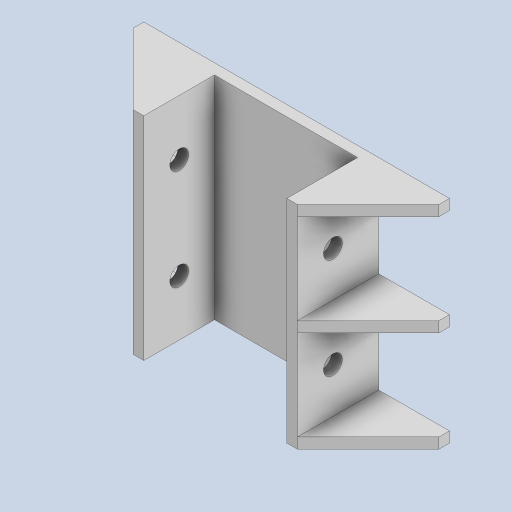
# Autodesk Inventor part: 2040 psu adapter
Saved by Autodesk Inventor 2024 (Build 280153000, 153)
## iProperties
Created: 2025-04-07
Part Number: 2040 psu adapter
Material: Generic
Document SubType Name: Modeling
Designer: jp.reyesf
Density: 1 g/cm^3
Appearance: Default
Author: jp.reyesf
Autodesk Inventor part; units mm, degrees
ref_plane "YZ Plane" through (0, 0, 0) normal (1, 0, 0) x (0, 1, 0)
ref_plane "XZ Plane" through (0, 0, 0) normal (0, 1, 0) x (-1, 0, 0)
ref_plane "XY Plane" through (0, 0, 0) normal (0, 0, 1) x (1, 0, 0)
sketch "Sketch1" plane through (0, 0, 0) normal (0, 1, 0) x (-1, 0, 0)
  line L0 (23.25, 0) -> (23.25, 23)
  line L1 (23.25, 23) -> (20.25, 23)
  line L2 (20.25, 23) -> (20.25, 3)
  line L3 (20.25, 3) -> (-20.25, 3)
  line L4 (-20.25, 3) -> (-20.25, 23)
  line L5 (-20.25, 23) -> (-23.25, 23)
  line L6 (-23.25, 23) -> (-23.25, 0)
  line L7 (-23.25, 0) -> (23.25, 0)
  line L8 (23.25, 23) -> (43.25, 3)
  line L9 (43.25, 3) -> (43.25, 0)
  line L10 (43.25, 0) -> (23.25, 0)
  line L11 (23.25, 0) -> (-23.25, 0)
  line L12 (-43.25, 0) -> (-43.25, 3)
  line L13 (-43.25, 3) -> (-23.25, 23)
  line L14 (-43.25, 0) -> (-23.25, 0)
  point P0 (0, 0)
  point P1 (0, 0)
  dimension "d0" = 20
  dimension "d1" = 40.5
  dimension "d2" = 3
  dimension "d3" = 3
  dimension "d13" = 45
  dimension "d14" = 45
  constraints: 31 end point, 7 perpendicular, 3 equal length, 3 point on line, 3 vertical, 1 coincident, 1 collinear, 1 horizontal, 1 midpoint
  measures "d0" distance of L1.end L2.end
  measures "d1" distance of L2.end L3.end
  measures "d2" distance between parallel lines of L7 L3
  measures "d3" distance of L0.end L1.end
  measures "d13" angle of L0 L8
  measures "d14" angle of L6 L13
extrude "Extrusion1" add sketch "Sketch1" along normal blind 60 contours L7 L6 L5 L4 L3 L2 L1 L0
extrude "Extrusion3" add sketch "Sketch1" along normal blind 3 contours L0 L8 L9 L10 | L14 L12 L13 L6
ref_plane "Work Plane1" through (0, 30, 0) normal (0, 1, 0) x (1, 0, 0)
pattern_linear "Rectangular Pattern1" count 3 spacing 28.5 along (0, 1, 0) of "Extrusion3"
sketch "Sketch4" plane through (0, 30, 0) normal (0, 1, 0) x (1, 0, 0)
  point P0 (0, 0)
sketch "Sketch5" plane through (-20.25, 0, 23) normal (1, 0, 0) x (0, 0, -1)
  line L0 (0, 57) -> (23, 57) projected
  line L1 (23, 31.5) -> (23, 57) projected
  line L2 (23, 31.5) -> (0, 31.5) projected
  line L3 (0, 31.5) -> (0, 57) projected
  line L4 (0, 28.5) -> (23, 28.5) projected
  line L5 (23, 3) -> (23, 28.5) projected
  line L6 (23, 3) -> (0, 3) projected
  line L7 (0, 3) -> (0, 28.5) projected
  line L8 (0, 0) -> (20, 0) projected
  line L9 (20, 0) -> (20, 60) projected
  line L10 (0, 60) -> (20, 60) projected
  line L11 (0, 0) -> (0, 60) projected
  line L12 (20, 57) -> (0, 31.5) construction
  line L13 (20, 28.5) -> (0, 3) construction
  circle A0 centre (10, 44.25) radius 2.65
  circle A1 centre (10, 15.75) radius 2.65
  point P0 (23, 0)
  dimension "d26" = 5.3
  dimension "d27" = 5.3
  constraints: 4 end point, 4 point on line, 2 centre point, 2 midpoint, 1 parallel
  measures "d26" diameter of A0
  measures "d27" diameter of A1
extrude "Extrusion5" cut sketch "Sketch5" along normal through all both and the other way through all contours A0 | A1
body "Solid1"
